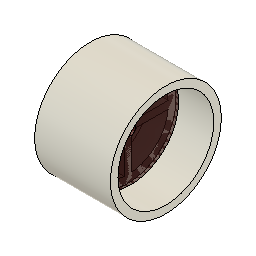
check valve v2 (Autodesk Fusion 360 design; units mm, degrees)
Autodesk Fusion 360 part; units mm, degrees
note: some values were not read from the file. Set by a fixed rule: which sketch regions a step uses.
sketch "Sketch1" plane through (0, 0, 0) normal (1, 0, 0) x (0, 0, -1)
  circle A0 centre (0, 0) radius 12.65
  circle A1 centre (0, 0) radius 14.65
  line L0 (0, 0) -> (0, 12.65) construction
  line L1 (0, 0) -> (0, -12.65) construction
  line L2 (-1, 12.6104) -> (-1, -12.6104)
  line L3 (1, 12.6104) -> (1, -12.6104)
  line L4 (0, 0) -> (12.65, 0) construction
  line L5 (0, 0) -> (-12.65, 0) construction
  line L6 (12.6104, -1) -> (-12.6104, -1)
  line L7 (-12.6104, 1) -> (12.6104, 1)
  circle A2 centre (0, 0) radius 2.5
  circle A3 centre (0, 0) radius 10.65
  circle A4 centre (0, 0) radius 1.3894
  dimension "d1" = 25.3
  dimension "d2" = 2
  dimension "d3" = 2
  dimension "d4" = 2
  dimension "d5" = 5
  dimension "d6" = 2
  dimension "d7" = 2.7788
  constraint coincident A0.centre A1.centre
  constraint coincident A0 L0.end
  constraint vertical L0
  constraint parallel L0 L1
  constraint coincident A0 L1.end
  constraint coincident A0 L2.start
  constraint coincident A0 L2.end
  constraint parallel L0 L2
  constraint coincident A0 L3.start
  constraint coincident A0 L3.end
  constraint parallel L1 L3
  constraint symmetric L0 L2 L3
  constraint perpendicular L3 L4
  constraint perpendicular L0 L5
  constraint coincident A0 L5.end
  constraint coincident A0 L4.end
  constraint coincident A0 L6.start
  constraint coincident A0 L6.end
  constraint perpendicular L1 L6
  constraint coincident A0 L7.start
  constraint coincident A0 L7.end
  constraint perpendicular L0 L7
  constraint symmetric L4 L6 L7
  constraint concentric A0 A2
  constraint concentric A1 A4
  measures "d1" diameter of A0
  measures "d2" distance of A0 A1
  measures "d3" distance of L2 L3
  measures "d4" distance of L6 L7
  measures "d5" diameter of A2
  measures "d6" distance of A0 A3
  measures "d7" diameter of A4
extrude "Extrude1" add sketch "Sketch1" along normal mid plane 20 makes body 1
extrude "Extrude2" add sketch "Sketch1" against normal blind 5 contours A0 L6 L7 A3 | A0 L3 L7 A3 | A0 L3 L6 A3 | A0 L2 L3 A3 | L6 L7 A2 A3 | A0 L2 L3 A3 | A0 L2 L7 A3 | L2 L3 A2 A3 | L3 L6 L7 A2 A4 | L3 L7 A2 | A0 L2 L6 A3 | L2 L3 A2 A3 | L3 L6 A2 | A0 L6 L7 A3 | L2 L3 L7 A2 A4 | L3 L7 A4 | L2 L3 L6 A2 A4 | L3 L6 A4 | L6 L7 A2 A3 | L2 L7 A2 | L2 L6 A2 | L2 L6 L7 A2 A4 | L2 L7 A4 | L2 L6 A4 bodies 1
sketch "Sketch2" plane through (0, 0, 0) normal (1, 0, 0) x (0, 0, -1)
  circle A0 centre (0, 0) radius 1.3894
  arc A1 (-10.6029, -1) -> (-1, -10.6029) centre (0, 0) ccw
  line L0 (-10.6029, -1) -> (-2.2913, -1)
  arc A2 (-2.2913, -1) -> (-1, -2.2913) centre (0, 0) ccw
  line L1 (-1, -2.2913) -> (-1, -10.6029)
  line L2 (10.6029, 1) -> (2.2913, 1)
  arc A3 (2.2913, 1) -> (1, 2.2913) centre (0, 0) ccw
  line L3 (1, 2.2913) -> (1, 10.6029)
  arc A4 (10.6029, 1) -> (1, 10.6029) centre (0, 0) ccw
  line L4 (1, -10.6029) -> (1, -2.2913)
  arc A5 (1, -2.2913) -> (2.2913, -1) centre (0, 0) ccw
  line L5 (2.2913, -1) -> (10.6029, -1)
  arc A6 (1, -10.6029) -> (10.6029, -1) centre (0, 0) ccw
  line L6 (-2.2913, 1) -> (-10.6029, 1)
  arc A7 (-1, 10.6029) -> (-10.6029, 1) centre (0, 0) ccw
  line L7 (-1, 10.6029) -> (-1, 2.2913)
  arc A8 (-1, 2.2913) -> (-2.2913, 1) centre (0, 0) ccw
  circle A9 centre (0, 0) radius 12.65
extrude "Extrude1'" add sketch "Sketch2" along normal blind 0.71 separate body contours A1 L0 A2 L1 | L2 A3 L3 A4 | L4 A5 L5 A6 | L6 A7 L7 A8 | A9 makes body 2 in component "Component"
component "Component" placed x (1, 0, 0) y (0, 1, 0) z (0, 0, 1) at (0, 0, 0)
